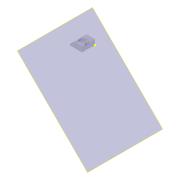
# Autodesk Inventor part: 00_KES400_DichroicMirror
Saved by Autodesk Inventor 2019.4 (Build 234330000, 330)
## iProperties
Created: 2020-06-28
Part Number: 00_KES400_DichroicMirror
Material: PMMA Plastic
Document SubType Name: Modeling
Designer: diederichbenedict
Density: 1.188 g/cm^3
Appearance: Polycarbonate - Clear
Author: diederichbenedict
Autodesk Inventor part; units mm, degrees
ref_plane "YZ Plane" through (0, 0, 0) normal (1, 0, 0) x (0, 1, 0)
ref_plane "XZ Plane" through (0, 0, 0) normal (0, 1, 0) x (-1, 0, 0)
ref_plane "XY Plane" through (0, 0, 0) normal (0, 0, 1) x (1, 0, 0)
sketch "Sketch1" plane through (0, 0, 0) normal (0, 0, 1) x (1, 0, 0)
  line L0 (0, 0) -> (-7.4, 0)
  line L1 (-7.4, 0) -> (-7.4, 3)
  line L2 (-7.4, 3) -> (0, 3)
  line L3 (0, 3) -> (0, 0)
  line L4 (-7.4, 0) -> (-7.4, 0.8)
  line L5 (-7.4, 0.8) -> (-5.2, 3)
  dimension "d0" = 7.4
  dimension "d1" = 3
  dimension "d3" = 135
  dimension "d11" = 2.2
  constraints: 12 end point, 2 parallel, 2 point on line, 1 horizontal, 1 perpendicular
  measures "d0" distance of L1.end L2.end
  measures "d1" distance of L0.end L1.end
  measures "d3" angle of L4 L5
  measures "d11" distance from line of L5.end L1
extrude "Extrusion1" add sketch "Sketch1" along normal blind 7.9 contours L0 L1 L5 L2 L3
sketch "Sketch2" plane through (-7.4, 0, 0) normal (0, -1, 0) x (1, 0, 0)
  line L0 (0, 0) -> (7.4, 0) projected
  line L1 (7.4, 0) -> (7.4, 7.9) projected
  line L2 (0, 7.9) -> (7.4, 7.9) projected
  line L3 (0, 0) -> (0, 7.9) projected
  circle A0 centre (3.7, 3.95) radius 1.5
  dimension "d6" = 3
  constraints: 1 centre point
  measures "d6" diameter of A0
extrude "Extrusion2" cut sketch "Sketch2" against normal blind 7.9 contours A0
sketch "Sketch3" plane through (-7.4, 0, 0) normal (0, -1, 0) x (1, 0, 0)
  point P0 (7.4, 0)
ref_plane "Work Plane1" through (-15.6286, 1.0607, 21.7368) normal (-0.7071, -0.7071, 0) x (0.7071, -0.7071, 0)
sketch "Sketch4" plane through (-15.6286, 1.0607, 21.7368) normal (-0.7071, -0.7071, 0) x (0.7071, -0.7071, 0)
  ellipse E0 centre (9.1848, -17.7868) end of major axis (9.1848, -16.2868) minor radius 1.0607 construction
  line L0 (6.5685, -21.7368) -> (11.8011, -21.7368) projected
  line L1 (11.8011, -21.7368) -> (11.8011, -13.8368) projected
  line L2 (6.5685, -13.8368) -> (11.8011, -13.8368) projected
  line L3 (6.5685, -21.7368) -> (6.5685, -13.8368) projected
  ellipse E1 centre (9.1848, -17.7868) end of major axis (9.1848, -16.2868) minor radius 1.0607 construction
  circle A0 centre (9.1848, -17.7868) radius 1.5 construction
  circle A1 centre (8.2455, -17.7868) radius 1.5374
  constraints: 2 centre point, 1 coincident, 3 other
extrude "Extrusion3" cut sketch "Sketch4" against normal through all contours A1
body "Solid1"
